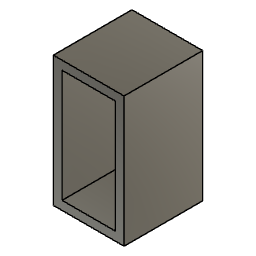
ServoMotorEnclosure (Autodesk Fusion 360 design; units mm, degrees)
Autodesk Fusion 360 part; units mm, degrees
sketch "Sketch1" plane through (0, 0, 0) normal (0, 1, 0) x (1, 0, 0)
  line L0 (0, 0) -> (16.2, 0)
  line L1 (16.2, 0) -> (16.2, -29.8)
  line L2 (16.2, -29.8) -> (0, -29.8)
  line L3 (0, -29.8) -> (0, 0)
  dimension "d1" = 16.2
  dimension "d2" = 29.8
  constraint horizontal L0
  constraint vertical L1
  constraint horizontal L2
  constraint vertical L3
  constraint coincident L0.start L3.end
  measures "d1" distance of L0.start L0.end
  measures "d2" distance of L0.start L2.end
extrude "Extrude1" add sketch "Sketch1" along normal blind 18
sketch "Sketch2" plane through (0, 0, 0) normal (0, -1, 0) x (1, 0, 0)
  line L0 (16.2, 29.8) -> (0, 29.8)
  line L1 (0, 29.8) -> (0, 0)
  line L2 (0, 0) -> (16.2, 0)
  line L3 (16.2, 0) -> (16.2, 29.8)
  line L4 (0, 29.8) -> (2, 29.8)
  line L5 (2, 29.8) -> (2, 27.8)
  line L6 (2, 27.8) -> (14.2, 27.8)
  line L7 (14.2, 27.8) -> (14.2, 2)
  line L8 (14.2, 2) -> (2, 2)
  line L9 (2, 2) -> (2, 27.8)
  dimension "d5" = 2
  dimension "d6" = 2
  dimension "d7" = 12.2
  dimension "d8" = 25.8
  constraint coincident L0.end L1.start
  constraint perpendicular L1 L4
  constraint perpendicular L4 L5
  constraint horizontal L6
  constraint vertical L7
  constraint horizontal L8
  constraint vertical L9
  measures "d5" distance of L0.end L4.end
  measures "d6" distance of L4.end L5.end
  measures "d7" distance of L5.end L6.end
  measures "d8" distance of L5.end L8.end
extrude "Extrude2" cut sketch "Sketch2" against normal blind 15 contours L6 L7 L8 L9
